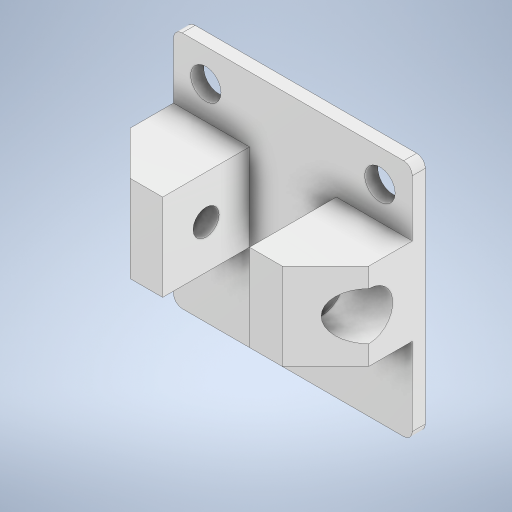
# Autodesk Inventor part: Gantry Plate
Saved by Autodesk Inventor 2023 (Build 270158000, 158)
## iProperties
Created: 2023-04-10
Part Number: Gantry Plate
Material: PC/ABS Plastic
Document SubType Name: Modeling
Designer: ethan
Density: 0.357273 g/cm^3
Appearance: Smooth - White
Author: ethan
Autodesk Inventor part; units mm, degrees
ref_plane "YZ Plane" through (0, 0, 0) normal (1, 0, 0) x (0, 1, 0)
ref_plane "XZ Plane" through (0, 0, 0) normal (0, 1, 0) x (-1, 0, 0)
ref_plane "XY Plane" through (0, 0, 0) normal (0, 0, 1) x (1, 0, 0)
sketch "Sketch1" plane through (0, 0, 0) normal (0, 1, 0) x (-1, 0, 0)
  line L0 (0, 0) -> (55, 0)
  line L1 (55, 0) -> (55, -55)
  line L2 (55, -55) -> (0, -55)
  line L3 (0, -55) -> (0, 0)
  line L4 (47.55, -7.45) -> (7.45, -7.45) construction
  line L5 (7.45, -7.45) -> (7.45, -47.55) construction
  line L6 (7.45, -47.55) -> (47.55, -47.55) construction
  line L7 (47.55, -47.55) -> (47.55, -7.45) construction
  circle A0 centre (47.55, -7.45) radius 3.5
  circle A1 centre (47.55, -47.55) radius 3.5
  circle A2 centre (7.45, -47.55) radius 3.5
  circle A3 centre (7.45, -7.45) radius 3.5
  circle A4 centre (47.55, -7.45) radius 12.5 construction
  circle A5 centre (27.5, -7.45) radius 3.5
  dimension "d0" = 55
  dimension "d1" = 55
  dimension "d2" = 40.1
  dimension "d3" = 40.1
  dimension "d4" = 7
  dimension "d5" = 7
  dimension "d6" = 7
  dimension "d7" = 7
  dimension "d8" = 7.45
  dimension "d9" = 7.45
  dimension "d13" = 25
  dimension "d14" = 7
  constraints: 16 end point, 6 centre point, 5 coincident, 4 parallel, 2 horizontal, 2 perpendicular, 1 midpoint
  measures "d0" distance of L1.end L2.end
  measures "d1" distance of L0.end L1.end
  measures "d2" distance of L6.end L5.end
  measures "d3" distance of L5.end L4.end
  measures "d4" diameter of A0
  measures "d5" diameter of A3
  measures "d6" diameter of A1
  measures "d7" diameter of A2
  measures "d8" distance between parallel lines of L1 L7
  measures "d9" distance from line of L2 L5.end
  measures "d13" diameter of A4
  measures "d14" diameter of A5
extrude "Extrusion1" add sketch "Sketch1" along normal blind 3 contours L0 L1 L2 L3 | A0 | A3
fillet "Fillet1" radius 2 4 edges at (-55, 1.5, 0) (0, 1.5, 0) (-55, 1.5, -55) (0, 1.5, -55)
sketch "Sketch2" plane through (0, 0, 0) normal (0, -1, 0) x (1, 0, 0)
  line L0 (-17.5, -40) -> (-37.5, -40) construction
  line L1 (-37.5, -40) -> (-37.5, -20) construction
  line L2 (-37.5, -20) -> (-17.5, -20) construction
  line L3 (-17.5, -20) -> (-17.5, -40) construction
  line L4 (-17.5, -20) -> (-37.5, -20)
  line L5 (-37.5, -20) -> (-37.5, 0)
  line L6 (-37.5, 0) -> (-17.5, 0)
  line L7 (-17.5, 0) -> (-17.5, -20)
  line L8 (-2, -55) -> (-53, -55) construction
  line L9 (-53, 0) -> (-2, 0) projected
  line L10 (0, -2) -> (0, -53) projected
  line L11 (-17.5, -20) -> (0, -20)
  line L12 (0, -20) -> (0, -40)
  line L13 (0, -40) -> (-17.5, -40)
  line L14 (-17.5, -40) -> (-17.5, -20)
  line L15 (-55, -53) -> (-55, -2) projected
  line L16 (-37.5, -20) -> (-55, -20)
  line L17 (-55, -20) -> (-55, -40)
  line L18 (-55, -40) -> (-37.5, -40)
  line L19 (-37.5, -40) -> (-37.5, -20)
  line L20 (0, -20) -> (-17.5, 0)
  line L21 (-37.5, 0) -> (-55, -20)
  point P0 (0, 0)
  point P1 (0, -20)
  point P2 (0, -20)
  dimension "d15" = 20
  dimension "d16" = 20
  dimension "d17" = 20
  dimension "d18" = 51
  dimension "d19" = 15.5
  constraints: 36 end point, 8 parallel, 4 horizontal, 4 perpendicular, 3 point on line, 1 collinear
  measures "d15" distance of L1.end L2.end
  measures "d16" distance of L0.end L1.end
  measures "d17" distance of L4.end L5.end
  measures "d18" distance of L8.start L8.end
  measures "d19" distance from line of L8.start L3
extrude "Extrusion8" add sketch "Sketch2" along normal blind 20 contours L11 L10 L13 L14 | L19 L18 L15 L16
sketch "Sketch6" plane through (-55, 0, -53) normal (-1, 0, 0) x (0, 0, 1)
  line L0 (13, -20) -> (33, -20) construction
  line L1 (13, 0) -> (33, 0) construction
  line L2 (13, -20) -> (33, 0) construction
  circle A0 centre (23, -10) radius 3
  point P0 (53, 0)
  dimension "d44" = 6
  constraints: 2 end point, 1 centre point, 1 midpoint
  measures "d44" diameter of A0
extrude "Extrusion9" cut sketch "Sketch6" against normal through all
sketch "Sketch7" plane through (-55, 0, -53) normal (-1, 0, 0) x (0, 0, 1)
  circle A0 centre (23, -10) radius 3 projected
  circle A1 centre (23, -10) radius 5.5
  point P0 (53, 0)
  dimension "d47" = 11
  constraints: 1 centre point, 1 coincident
  measures "d47" diameter of A1
extrude "Extrusion10" cut sketch "Sketch7" against normal blind 11 contours A0 | A1
sketch "Sketch8" plane through (0, 0, -53) normal (1, 0, 0) x (0, 0, -1)
  line L0 (-33, 0) -> (-33, -20) construction
  line L1 (-13, 0) -> (-33, 0) construction
  line L2 (-33, -20) -> (-13, 0) construction
  circle A0 centre (-23, -10) radius 5.5 projected
  circle A1 centre (-23, -10) radius 5.5 construction
  point P0 (-53, 0)
  constraints: 2 end point, 1 centre point, 1 coincident
extrude "Extrusion11" cut sketch "Sketch8" against normal blind 11
chamfer "Chamfer3" distance 10 angle 45 2 edges at (0, -20, -30) (-55, -20, -30)
equation "\"d1\" = d0"
equation "\"d3\" = d2"
equation "\"d5\" = d4"
equation "\"d6\" = d4"
equation "\"d7\" = d4"
equation "\"d8\" = -0.5 * d2 + 0.5 * d0"
equation "\"d9\" = -0.5 * d3 + 0.5 * d1"
equation "\"d14\" = d4"
equation "\"d19\" = -0.5 * d15 + 0.5 * d18"
body "Solid1"
